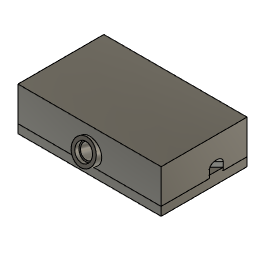
Fluorescence cell rev3 v5 (Autodesk Fusion 360 design; units mm, degrees)
Autodesk Fusion 360 part; units mm, degrees
sketch "Sketch2" plane through (0, 0, 0) normal (0, 0, 1) x (1, 0, 0) in component "Base"
  line L0 (0, 0) -> (0, 50)
  line L1 (0, 0) -> (25, 0)
  line L2 (25, 0) -> (25, 30)
  line L3 (25, 30) -> (0, 30)
  line L4 (0, 0) -> (-25, 0)
  line L5 (-25, 0) -> (-25, 30)
  line L6 (-25, 30) -> (0, 30)
  line L7 (0, 8) -> (7.5, 8) construction
  line L8 (18.1066, 12.3934) -> (25, 19.2868) construction
  arc A0 (7.5, 8) -> (18.1066, 12.3934) centre (7.5, 23) ccw construction
  line L9 (0, 6.3) -> (7.5, 6.3)
  arc A1 (7.5, 6.3) -> (19.3087, 11.1913) centre (7.5, 23) ccw
  line L10 (19.3087, 11.1913) -> (26.2021, 18.0847)
  line L11 (0, 9.7) -> (7.5, 9.7)
  arc A2 (7.5, 9.7) -> (16.9045, 13.5955) centre (7.5, 23) ccw
  line L12 (16.9045, 13.5955) -> (23.7979, 20.4889)
  line L13 (23.7979, 20.4889) -> (27.2239, 23.9148)
  line L14 (0, 9.7) -> (-7.5, 9.7)
  arc A3 (-16.9045, 13.5955) -> (-7.5, 9.7) centre (-7.5, 23) ccw
  line L15 (-16.9045, 13.5955) -> (-23.7979, 20.4889)
  line L16 (-23.7979, 20.4889) -> (-27.2239, 23.9148)
  line L17 (0, 6.3) -> (-7.5, 6.3)
  line L18 (-19.3087, 11.1913) -> (-26.2021, 18.0847)
  arc A4 (-19.3087, 11.1913) -> (-7.5, 6.3) centre (-7.5, 23) ccw
  dimension "d1" = 50
  dimension "d2" = 25
  dimension "d3" = 30
  dimension "d31" = 8
  dimension "d32" = 45
  dimension "d33" = 15
  dimension "d34" = 15
  dimension "d35" = 1.7
  dimension "d36" = -1.7
  constraint coincident L0.start L1.start
  constraint vertical L0
  constraint horizontal L1
  constraint perpendicular L1 L2
  constraint coincident L0 L3.end
  constraint perpendicular L0 L3
  constraint coincident L0 L7.start
  constraint perpendicular L0 L7
  constraint coincident L2 L8.end
  constraint tangent L7 A0
  constraint tangent L8 A0
  constraint parallel L12 L13
  constraint symmetric L0 L9.start L17.start
  constraint symmetric L0 L9.end L17.end
  constraint symmetric L0 A1.end L18.start
  constraint symmetric L0 A1 A4
  constraint symmetric L0 L10.end L18.end
  constraint symmetric L0 L11.start L14.start
  constraint symmetric L0 L11.end L14.end
  constraint symmetric L0 A2.end A3.start
  constraint symmetric L0 A2 A3
  constraint symmetric L0 L12.end L15.end
  constraint symmetric L0 L13.end L16.end
  measures "d1" distance of L0.start L0.end
  measures "d2" distance of L0.start L1.end
  measures "d3" distance of L1.end L2.end
  measures "d31" distance of L1 L7.start
  measures "d32" angle of L7 L8
  measures "d33" radius of A0
extrude "Extrude1" add sketch "Sketch2" along normal blind 12 makes body 1 in component "Base"
extrude "Extrude2" cut sketch "Sketch2" along normal blind 4.4 contours L0 L5 L14 A3 L15 L16 L17 L18 A4 | L0 L2 L9 A1 L10 L11 A2 L12 L13 bodies 1 in component "Base"
fillet "Fillet1" radius 1.7 10 edges at (-22.1543, 14.037, 4.4) (-13.8908, 7.5712, 4.4) (0, 6.3, 4.4) (13.8908, 7.5712, 4.4) (22.1543, 14.037, 4.4) (20.9523, 17.6432, 4.4) (12.5897, 10.7124, 4.4) (0, 9.7, 4.4) (-12.5897, 10.7124, 4.4) (-20.9523, 17.6432, 4.4) on bodies 1 in component "Base"
sketch "Sketch1" plane through (0, 0, 0) normal (0, 0, 1) x (1, 0, 0) in component "light_sensor"
  line L0 (0, 0) -> (7.8, 0)
  line L1 (7.8, 0) -> (7.8, -10.7)
  line L2 (7.8, -10.7) -> (0, -10.7)
  line L3 (0, -10.7) -> (0, 0)
  circle A0 centre (3.9, -8.2) radius 1
  line L4 (3.9, -10.7) -> (3.9, -8.2) construction
  line L5 (1.3, -5.4) -> (2.8, -5.4)
  line L6 (2.8, -5.4) -> (2.8, -4.4)
  line L7 (2.8, -4.4) -> (1.3, -4.4)
  line L8 (1.3, -4.4) -> (1.3, -5.4)
  dimension "d15" = 7.8
  dimension "d16" = 10.7
  dimension "d17" = 2
  dimension "d18" = 2.5
  dimension "d19" = 1
  dimension "d20" = 1.5
  dimension "d21" = 6.3
  dimension "d52" = 1.3
  constraint horizontal L0
  constraint vertical L1
  constraint horizontal L2
  constraint vertical L3
  constraint coincident L0.start L3.end
  constraint midpoint L2 L4.start
  constraint coincident A0.centre L4.end
  constraint vertical L4
  constraint horizontal L5
  constraint vertical L6
  constraint horizontal L7
  constraint vertical L8
  measures "d15" distance of L1.end L2.end
  measures "d16" distance of L0.start L2.end
  measures "d17" diameter of A0
  measures "d18" distance of L2 A0.centre
  measures "d19" distance of L5.start L7.end
  measures "d20" distance of L6.end L7.end
  measures "d21" distance of L2 L7
  measures "d52" distance of L3 L8
extrude "Extrude1'" add sketch "Sketch1" against normal blind 1.6 separate body contours L0 L1 L2 L3 | L5 L6 L7 L8 makes body 2 in component "light_sensor"
extrude "Extrude2'" add sketch "Sketch1" along normal blind 0.8 contours L5 L6 L7 L8 bodies 2 in component "light_sensor"
ref_plane "WorkPlane1" through (-3.75, 8, 2.7) normal (0, 0.258819, 0.965926) x (1, 0, 0) in component "Base"
sketch "Sketch3" plane through (0, 0, 0) normal (0, -1, 0) x (1, 0, 0) in component "Base"
  line L0 (-25, 0) -> (25, 0)
  line L1 (25, 0) -> (25, 12)
  line L2 (25, 12) -> (-25, 12)
  line L3 (-25, 12) -> (-25, 0)
  line L4 (7.5, 2.7) -> (-7.5, 2.7) construction
  line L5 (-7.5, 2.7) -> (-7.5, 0) construction
  line L6 (-7.5, 0) -> (7.5, 0) construction
  line L7 (7.5, 0) -> (7.5, 2.7) construction
  line L8 (7.5, 2.7) -> (7.5, 4.4) construction
  line L9 (7.5, 2.7) -> (-7.5, 2.7) construction
  line L10 (-7.5, 2.7) -> (-7.5, 4.4) construction
  line L11 (-7.5, 2.7) -> (7.5, 2.7) construction
  line L12 (0, 2.7) -> (0, 5.2) construction
  dimension "d40" = 2.5
  constraint midpoint L11 L12.start
  constraint perpendicular L11 L12
  measures "d40" distance of L12.start L12.end
ref_plane "WorkPlane2" through (-1.875, 0, 4.8436) normal (0, -0.965926, 0.258819) x (-1, 0, 0) in component "Base"
sketch "Sketch4" plane through (-1.875, -0.1375, 4.3304) normal (0, -0.965926, 0.258819) x (-1, 0, 0) in component "Base"
  line L0 (-9.375, -0.9713) -> (5.625, -0.9713) construction
  line L1 (5.625, -0.9713) -> (5.625, 1.6367) construction
  line L2 (5.625, 1.6367) -> (-9.375, 1.6367) construction
  line L3 (-9.375, 1.6367) -> (-9.375, -0.9713) construction
  line L4 (-9.375, -0.0913) -> (-9.375, -2.2313) construction
  line L5 (-9.375, -0.0913) -> (5.625, -0.0913) construction
  line L6 (5.625, -0.0913) -> (5.625, -2.2313) construction
  line L7 (5.625, -0.9713) -> (-9.375, -0.9713) construction
  point P0 (-1.875, -0.0913)
  constraint midpoint L5 P0
hole "Hole1" at (0, -0.1139, 4.4186) direction (0, 0.965926, -0.258819) diameter 5 depth 7 tip angle 90 bodies 1 in component "Base"
hole "Hole1'" [no effect] in component "light_sensor"
hole "Hole2" at (0, -0.1139, 4.4186) direction (0, -0.965926, 0.258819) diameter 5 depth 5 tip angle 90 bodies 1 in component "Base"
sketch "Sketch1 (2)" plane through (0, 0, 0) normal (0, 1, 0) x (1, 0, 0) in component "LED 5mm"
  line L0 (0, 0) -> (0, -18)
  line L1 (0, 0) -> (2.95, 0)
  line L2 (2.95, 0) -> (2.95, -1)
  line L3 (2.95, -1) -> (2.5, -1)
  line L4 (2.5, -1) -> (2.5, -8.7)
  line L5 (2.5, -8.7) -> (0, -8.7)
  dimension "d53" = 8.7
  dimension "d54" = 1
  dimension "d55" = 5.9
  dimension "d56" = 5
  constraint coincident L0.start L1.start
  constraint vertical L0
  constraint perpendicular L0 L1
  constraint perpendicular L1 L2
  constraint perpendicular L2 L3
  constraint perpendicular L3 L4
  constraint coincident L0 L5.end
  constraint perpendicular L0 L5
  measures "d53" distance of L1 L5
  measures "d54" distance of L1.end L2.end
revolve "Revolve1" add sketch "Sketch1 (2)" angle 360 about axis through (0, 0, 0) along (0, 0, 1) separate body makes body 3 in component "LED 5mm"
fillet "Fillet1'" radius 2.5 1 edges at (-2.3308, -0.904, 8.7) on bodies 3 in component "LED 5mm"
sketch "Sketch1 (3)" plane through (0, 0, 0) normal (0, 0, -1) x (1, 0, 0) in component "Lid"
  line L0 (-25, -16.8826) -> (-19.3087, -11.1913)
  arc A0 (-7.5, -6.3) -> (-19.3087, -11.1913) centre (-7.5, -23) ccw
  line L1 (-7.5, -6.3) -> (7.5, -6.3)
  arc A1 (19.3087, -11.1913) -> (7.5, -6.3) centre (7.5, -23) ccw
  line L2 (19.3087, -11.1913) -> (25, -16.8826)
  line L3 (25, -16.8826) -> (25, 0)
  line L4 (25, 0) -> (-25, 0)
  line L5 (-25, 0) -> (-25, -16.8826)
  line L6 (-16.9045, -13.5955) -> (-25, -21.691)
  line L7 (-25, -21.691) -> (-25, -30) construction
  line L8 (-25, -30) -> (25, -30) construction
  line L9 (25, -30) -> (25, -21.691) construction
  line L10 (25, -21.691) -> (16.9045, -13.5955)
  arc A2 (16.9045, -13.5955) -> (7.5, -9.7) centre (7.5, -23) ccw
  line L11 (7.5, -9.7) -> (-7.5, -9.7)
  arc A3 (-7.5, -9.7) -> (-16.9045, -13.5955) centre (-7.5, -23) ccw
  circle A4 centre (1.85, -5.0146) radius 1 construction
  line L12 (5.75, -2.5146) -> (-2.05, -2.5146) construction
  line L13 (-2.05, -2.5146) -> (-2.05, -13.2146) construction
  line L14 (-2.05, -13.2146) -> (5.75, -13.2146) construction
  line L15 (5.75, -13.2146) -> (5.75, -2.5146) construction
  line L16 (-25, 0) -> (25, 0)
  line L17 (25, 0) -> (25, -30)
  line L18 (25, -30) -> (-25, -30)
  line L19 (-25, -30) -> (-25, 0)
  line L20 (-2.05, -2.5146) -> (5.75, -2.5146)
  line L21 (5.75, -2.5146) -> (5.75, -13.2146)
  line L22 (5.75, -13.2146) -> (-2.05, -13.2146)
  line L23 (-2.05, -13.2146) -> (-2.05, -2.5146)
  line L24 (-2.05, -10.7146) -> (5.75, -10.7146)
  line L25 (21, -26) -> (-21, -26) construction
  line L26 (-21, -26) -> (-21, -4) construction
  line L27 (-21, -4) -> (21, -4) construction
  line L28 (21, -4) -> (21, -26) construction
  point P0 (-21, -4)
  point P1 (21, -4)
  point P2 (21, -26)
  point P3 (-21, -26)
  dimension "d68" = 2.5
  dimension "d73" = 4
  constraint horizontal L16
  constraint vertical L17
  constraint horizontal L18
  constraint vertical L19
  constraint coincident L8.end L9.start
  constraint coincident L4.end L5.start
  constraint horizontal L20
  constraint vertical L21
  constraint horizontal L22
  constraint vertical L23
  constraint coincident L14.end L15.start
  constraint coincident L12.end L13.start
  constraint coincident L13 L24.start
  constraint coincident L21 L24.end
  constraint perpendicular L21 L24
  constraint coincident P0 L26.end
  constraint coincident P1 L27.end
  constraint coincident P2 L25.start
  constraint coincident P3 L25.end
  measures "d68" distance of L22 L24
extrude "Extrude1''" add sketch "Sketch1 (3)" along normal blind 3 separate body makes body 4 in component "Lid"
extrude "Extrude2''" add sketch "Sketch1 (3)" against normal blind 1 contours L0 A0 L1 L6 L11 A3 L19 L23 | L1 A1 L2 L10 A2 L11 L17 L21 bodies 4 in component "Lid"
extrude "Extrude3" cut sketch "Sketch1 (3)" along normal blind 7 contours L21 L22 L23 L24 bodies 4 in component "Lid"
fillet "Fillet1''" radius 1 4 edges at (-2.05, 13.2146, -1.5) (5.75, 13.2146, -1.5) (-2.05, 10.7146, -1.5) (5.75, 10.7146, -1.5) on bodies 4 in component "Lid"
hole "Hole1''" at (-21, 4, 0) at (-21, 26, 0) at (21, 26, 0) at (21, 4, 0) direction (0, 0, -1) diameter 4 end through all bodies 4 in component "Lid"
hole "Hole3" at (-21, 26, 0) at (-21, 4, 0) at (21, 4, 0) at (21, 26, 0) direction (0, 0, 1) diameter 3.15 depth 10 tip angle 180 bodies 1 in component "Base"
sketch "Sketch5" plane through (0, 0, 0) normal (0, 0, -1) x (1, 0, 0) in component "Base"
  circle A0 centre (-21, -26) radius 1.575
  circle A1 centre (21, -26) radius 1.575
  line L0 (-16.9045, -13.5955) -> (-25, -21.691)
  line L1 (-25, -21.691) -> (-25, -30)
  line L2 (-25, -30) -> (25, -30)
  line L3 (25, -30) -> (25, -21.691)
  line L4 (25, -21.691) -> (16.9045, -13.5955)
  arc A2 (16.9045, -13.5955) -> (7.5, -9.7) centre (7.5, -23) ccw
  line L5 (7.5, -9.7) -> (-7.5, -9.7)
  arc A3 (-7.5, -9.7) -> (-16.9045, -13.5955) centre (-7.5, -23) ccw
  circle A4 centre (1.85, -5.0146) radius 1
  line L6 (5.75, -2.5146) -> (-2.05, -2.5146)
  line L7 (-2.05, -2.5146) -> (-2.05, -13.2146)
  line L8 (-2.05, -13.2146) -> (5.75, -13.2146)
  line L9 (5.75, -13.2146) -> (5.75, -2.5146)
extrude "Extrude3'" cut sketch "Sketch5" against normal blind 0.5 contours L5 L6 L7 L9 | L5 L7 L8 L9 | A4 bodies 1 in component "Base"
extrude "Extrude4" cut sketch "Sketch1 (3)" along normal blind 1.5 contours L1 L20 L21 L23 | L1 L11 L21 L23 | L11 L21 L23 L24 | L21 L22 L23 L24 bodies 4 in component "Lid"
sketch "Sketch6" plane through (-1.875, 0, 4.8436) normal (0, -0.965926, 0.258819) x (-1, 0, 0) in component "Base"
  circle A0 centre (-1.875, 0.44) radius 2.5 construction
  circle A1 centre (-1.875, 0.44) radius 2.5
  circle A2 centre (-1.875, 0.44) radius 4.25
  dimension "d84" = 5
  dimension "d85" = 8.5
  constraint concentric A0 A1
  constraint concentric A1 A2
  measures "d84" diameter of A1
  measures "d85" diameter of A2
extrude "Extrude4'" add sketch "Sketch6" along normal blind 2 and the other way blind 1 bodies 1 in component "Base"
ref_plane "WorkPlane3" through (-1.875, -0.483, 4.973) normal (0, -0.965926, 0.258819) x (-1, 0, 0) in component "Base"
sketch "Sketch7" plane through (-1.875, -0.483, 4.973) normal (0, -0.965926, 0.258819) x (-1, 0, 0) in component "Base"
  circle A0 centre (-1.875, 0.44) radius 2.95 construction
  circle A1 centre (-1.875, 0.44) radius 3
  dimension "d91" = 6
  constraint concentric A0 A1
  measures "d91" diameter of A1
extrude "Extrude5" cut sketch "Sketch7" along normal blind 4.5 bodies 1 in component "Base"
extrude "Extrude5'" cut 3 faces at (0.8833, 5.248, -1.5) (5.5535, 13.0182, -1.5) (-1.8535, 13.0182, -1.5) along direction (0, 0, -1) blind 0.3 on bodies 4 bodies 4 in component "Lid"
component "Base" placed x (1, 0, 0) y (0, 1, 0) z (0, 0, 1) at (0, 0, 0)
component "light_sensor" placed x (1, 0, 0) y (0, 1, 0) z (0, 0, 1) at (-2.05, 13.2146, 0)
component "LED 5mm" placed x (1, 0, 0) y (0, -0.258819, -0.965926) z (0, 0.965926, -0.258819) at (0, -1.7548, 4.8583)
component "Lid" placed x (1, 0, 0) y (0, 1, 0) z (0, 0, 1) at (0, 0, 0)
equation "tube = 3.4 mm"
equation "d11 = tube + 1 mm"
equation "d35 = tube / 2"
equation "d36 = -tube / 2"
equation "d38 = tube / 2"
